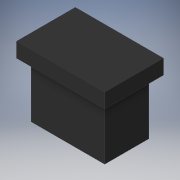
# Autodesk Inventor part: switch
Saved by Autodesk Inventor 2019 (Build 230136000, 136)
## iProperties
Created: 2019-02-16
Part Number: switch
Material: Generic
Document SubType Name: Modeling
Designer: suchanek
Density: 1 g/cm^3
Appearance: Default
Author: suchanek
Autodesk Inventor part; units mm, degrees
ref_plane "YZ Plane" through (0, 0, 0) normal (1, 0, 0) x (0, 1, 0)
ref_plane "XZ Plane" through (0, 0, 0) normal (0, 1, 0) x (-1, 0, 0)
ref_plane "XY Plane" through (0, 0, 0) normal (0, 0, 1) x (1, 0, 0)
sketch "Sketch1" plane through (0, 0, 0) normal (0, 1, 0) x (-1, 0, 0)
  line L0 (-10, 6) -> (10, 6)
  line L1 (10, 6) -> (10, -6)
  line L2 (10, -6) -> (-10, -6)
  line L3 (-10, -6) -> (-10, 6)
  line L4 (-10, 6) -> (10, -6) construction
  line L5 (10, 6) -> (-10, -6) construction
  point P0 (0, 0)
  dimension "d0" = 20
  dimension "d1" = 12
  constraints: 12 end point, 2 midpoint, 2 parallel, 1 horizontal, 1 perpendicular
  measures "d0" distance of L1.end L2.end
  measures "d1" distance of L0.end L1.end
extrude "Extrusion1" add sketch "Sketch1" along normal blind 15
sketch "Sketch2" plane through (0, 15, 0) normal (0, 1, 0) x (1, 0, 0)
  line L0 (12, -8) -> (-12, -8)
  line L1 (-12, -8) -> (-12, 8)
  line L2 (-12, 8) -> (12, 8)
  line L3 (12, 8) -> (12, -8)
  line L4 (12, -8) -> (-12, 8) construction
  line L5 (-12, -8) -> (12, 8) construction
  line L6 (10, 6) -> (-10, 6) projected
  line L7 (-10, 6) -> (-10, -6) projected
  point P0 (0, 0)
  dimension "d4" = 2
  dimension "d5" = 2
  constraints: 12 end point, 2 midpoint, 2 parallel, 1 horizontal, 1 perpendicular
  measures "d4" distance between parallel lines of L2 L6
  measures "d5" distance between parallel lines of L7 L1
extrude "Extrusion2" add sketch "Sketch2" along normal blind 4
body "Solid1"
